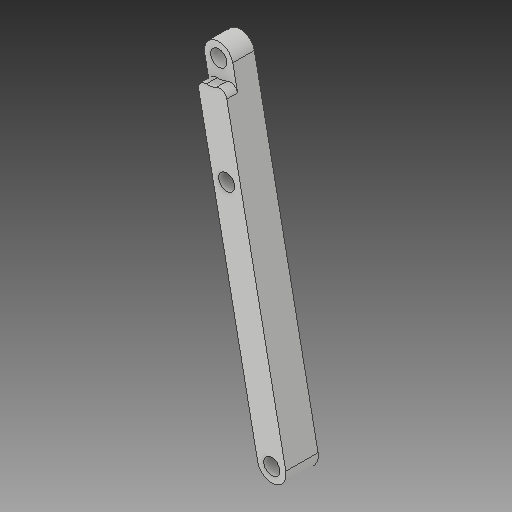
# Autodesk Inventor part: MasiveBone1
Saved by Autodesk Inventor 2017 (Build 210142000, 142)
## iProperties
Created: 2020-09-06
Part Number: MasiveBone1
Material: Generic
Document SubType Name: Modeling
Designer: agustin
Density: 1 g/cm^3
Appearance: Default
Author: agustin
Autodesk Inventor part; units mm, degrees
ref_plane "YZ Plane" through (0, 0, 0) normal (1, 0, 0) x (0, 1, 0)
ref_plane "XZ Plane" through (0, 0, 0) normal (0, 1, 0) x (-1, 0, 0)
ref_plane "XY Plane" through (0, 0, 0) normal (0, 0, 1) x (1, 0, 0)
sketch "Sketch1" plane through (0, 0, 0) normal (0, 0, 1) x (1, 0, 0)
  circle A0 centre (-4.5939, 35.2781) radius 2.25 projected
  circle A1 centre (-17.1487, 97.6266) radius 2.25 projected
  circle A2 centre (-22.3601, 123.5071) radius 2.25 projected
  line L0 (-4.5939, 35.2781) -> (-22.3601, 123.5071) construction
  line L1 (-0.6726, 36.0677) -> (-18.4388, 124.2967)
  line L2 (-26.2814, 122.7175) -> (-8.5151, 34.4885)
  arc A3 (-8.5151, 34.4885) -> (-0.6726, 36.0677) centre (-4.5939, 35.2781) ccw
  arc A4 (-18.4388, 124.2967) -> (-26.2814, 122.7175) centre (-22.3601, 123.5071) ccw
  point P0 (0, 0)
  point P1 (-13.477, 79.3926)
  dimension "d0" = 8
  constraints: 8 end point, 4 point on circle, 4 tangent, 2 centre point, 1 midpoint, 1 parallel
  measures "d0" diameter of A4
extrude "Extrusion1" add sketch "Sketch1" along normal blind 9
sketch "Sketch2" plane through (0, 0, 9) normal (0, 0, 1) x (1, 0, 0)
  circle A0 centre (-22.3601, 123.5071) radius 2.25 projected
  circle A1 centre (-22.3601, 123.5071) radius 5
  point P0 (0, 0)
  dimension "d3" = 10
  constraints: 1 centre point, 1 coincident
  measures "d3" diameter of A1
extrude "Extrusion2" cut sketch "Sketch2" against normal blind 3
fillet "Fillet1" radius 2 2 edges at (-25.6892, 119.7766, 7.5) (-17.8466, 121.3558, 7.5)
scale "Scale1" factors (0.5, 0.5, 0.5) then translate (-8.6991, 39.3015, 2.25) bodies 1
body "Solid1"
